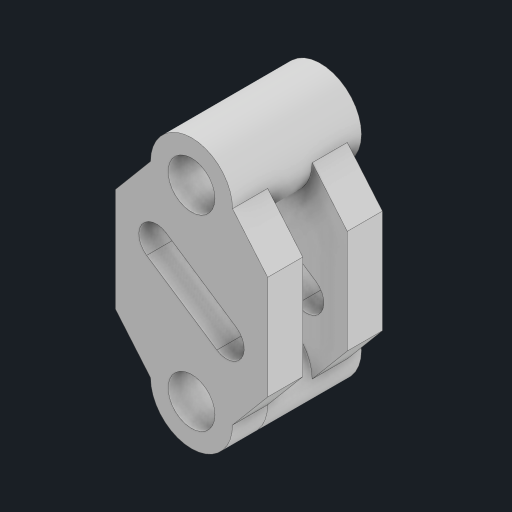
# Autodesk Inventor part: PotentiometerBracket
Saved by Autodesk Inventor 2023 (Build 270158000, 158)
## iProperties
Created: 2023-09-18
Part Number: PotentiometerBracket
Material: Generic
Document SubType Name: Modeling
Designer: valer
Density: 1 g/cm^3
Appearance: Default
Author: valer
Autodesk Inventor part; units mm, degrees
ref_plane "YZ Plane" through (0, 0, 0) normal (1, 0, 0) x (0, 1, 0)
sketch "Base" plane through (0, 0, 0) normal (0, 0, 1) x (1, 0, 0)
  circle A0 centre (16, -8) radius 2
  circle A1 centre (16, 8) radius 2
  circle A2 centre (16, -8) radius 3.5
  circle A3 centre (16, 8) radius 3.5
  point P0 (0, 0)
  dimension "d40" = 7
  constraints: 4 centre point, 2 coincident, 1 equal radius, 4 other
  measures "d40" diameter of A2
ref_plane "TopPlane" through (16.8435, -4.86, 8.0094) normal (0, 0, 1) x (1, 0, 0)
ref_plane "TopReferencePlane" through (16.8435, -4.86, 6.0094) normal (0, 0, 1) x (1, 0, 0)
extrude "BaseFeature" add sketch "Base" along normal up to surface (8.0094 mm away)
sketch "Cap" plane through (16, -8, 8.0094) normal (0, 0, 1) x (1, 0, 0)
  circle A0 centre (0, 0) radius 3.5 construction
  line L0 (3.5, 0) -> (6.5, 3.5753)
  line L1 (6.5, 3.5753) -> (6.5, 12.4247)
  line L2 (6.5, 12.4247) -> (3.5, 16)
  circle A1 centre (0, 16) radius 3.5 construction
  line L3 (-3.5, 0) -> (-3.5, 16) construction
  line L4 (-3.5, 8) -> (6.5, 8) construction
  circle A2 centre (0, 16) radius 3.5 projected
  arc A3 (-3.5, 0) -> (3.5, 0) centre (0, 0) ccw
  arc A4 (3.5, 16) -> (-3.5, 16) centre (0, 16) ccw
  circle A5 centre (0, 0) radius 2
  circle A6 centre (0, 16) radius 2
  line L5 (0, 0) -> (0, 16) construction
  line L6 (-3.5, 0) -> (-6.5, 3.5753)
  line L7 (-6.5, 3.5753) -> (-6.5, 12.4247)
  line L8 (-6.5, 12.4247) -> (-3.5, 16)
  point P0 (-16, 8)
  point P1 (-3.5, 16)
  point P2 (-3.5, 0)
  dimension "d43" = 140
  dimension "d44" = 140
  dimension "d45" = 10
  constraints: 18 end point, 4 centre point, 4 point on circle, 4 symmetric about line, 4 vertical, 2 horizontal alignment, 2 midpoint, 2 tangent, 1 equal length, 1 perpendicular, 7 other
  measures "d43" angle of L1 L0
  measures "d44" angle of L2 L1
  measures "d45" distance between parallel lines of L3 L1
extrude "CapFeature" add sketch "Cap" along normal blind 3
ref_plane "BottomPlane" through (16.7486, 4.86, 4.2094) normal (0, 0, -1) x (-1, 0, 0)
ref_plane "BottomReferencePlane" through (16.7486, 4.86, 5.2094) normal (0, 0, -1) x (-1, 0, 0)
sketch "Bottom" plane through (16.7486, 4.86, 4.2094) normal (0, 0, -1) x (-1, 0, 0)
  arc A0 (4.2486, 3.14) -> (-2.7514, 3.14) centre (0.7486, 3.14) ccw projected
  line L0 (4.2486, 3.14) -> (7.2486, -0.4353) projected
  line L1 (7.2486, -0.4353) -> (7.2486, -9.2847) projected
  line L2 (7.2486, -9.2847) -> (4.2486, -12.86) projected
  arc A1 (-2.7514, -12.86) -> (4.2486, -12.86) centre (0.7486, -12.86) ccw projected
  line L3 (-2.7514, -12.86) -> (-5.7514, -9.2847) projected
  line L4 (-5.7514, -9.2847) -> (-5.7514, -0.4353) projected
  line L5 (-5.7514, -0.4353) -> (-2.7514, 3.14) projected
  circle A2 centre (0.7486, 3.14) radius 2 projected
  circle A3 centre (0.7486, -12.86) radius 2 projected
  point P0 (16.7486, -4.86)
extrude "BottomFeature" add sketch "Bottom" along normal blind 3 contours L0 L1 L2 A1 L3 L4 L5 A0 | A2 | A3
sketch "Sketch11" plane through (16, -8, 11.0094) normal (0, 0, 1) x (1, 0, 0)
  line L0 (-3, 10.1304) -> (3, 6.1304) construction
  line L1 (-3.8321, 8.8824) -> (2.1679, 4.8824)
  line L2 (3.8321, 7.3785) -> (-2.1679, 11.3785)
  arc A0 (-2.1679, 11.3785) -> (-3.8321, 8.8824) centre (-3, 10.1304) ccw
  arc A1 (2.1679, 4.8824) -> (3.8321, 7.3785) centre (3, 6.1304) ccw
  line L3 (-6.5, 12.4247) -> (-6.5, 3.5753) projected
  line L4 (6.5, 3.5753) -> (6.5, 12.4247) projected
  point P0 (-16, 8)
  point P1 (0, 8.1304)
  dimension "d52" = 3.5
  dimension "d53" = 3.5
  dimension "d54" = 1.5
  constraints: 8 end point, 4 point on circle, 4 tangent, 2 centre point, 1 midpoint, 1 parallel
  measures "d52" distance from line of L3 L0.start
  measures "d53" distance from line of L4 L0.end
  measures "d54" radius of A1
extrude "Extrusion10" cut sketch "Sketch11" against normal through all
equation "\"d44\" = d43"
equation "\"d53\" = d52"
body "Solid2"
